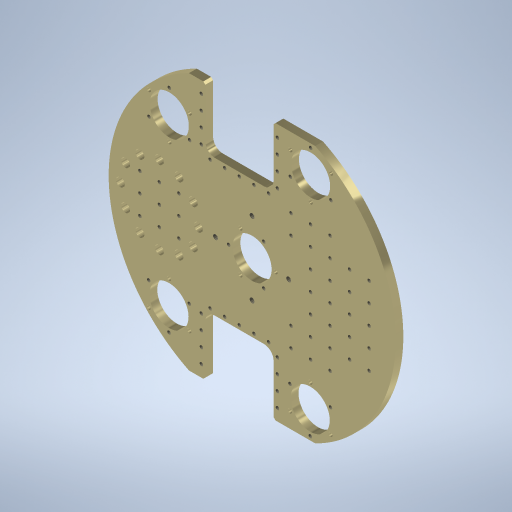
# Autodesk Inventor part: MXC_Plate_drawing
Saved by Autodesk Inventor 2024 (Build 280153000, 153)
## iProperties
Created: 2020-10-08
Part Number: MXC_Plate_drawing
Material: Generic
Document SubType Name: Modeling
Designer: mforsch
Density: 1 g/cm^3
Appearance: Default
Author: mforsch
Autodesk Inventor part; units mm, degrees
ref_plane "YZ Plane" through (0, 0, 0) normal (1, 0, 0) x (0, 1, 0)
ref_plane "XZ Plane" through (0, 0, 0) normal (0, 1, 0) x (-1, 0, 0)
ref_plane "XY Plane" through (0, 0, 0) normal (0, 0, 1) x (1, 0, 0)
sketch "Sketch1" plane through (0, 0, 0) normal (0, 0, 1) x (1, 0, 0)
  circle A0 centre (0, 0) radius 147
  dimension "d0" = 294
  constraints: 1 centre point, 1 coincident
  measures "d0" diameter of A0
extrude "Extrusion1" add sketch "Sketch1" along normal blind 8
sketch "Sketch2" plane through (0, 0, 8) normal (0, 0, 1) x (1, 0, 0)
  line L0 (-102.4138, 132) -> (116.069, 132)
  line L1 (116.069, 132) -> (116.069, 183.5862)
  line L2 (116.069, 183.5862) -> (-102.4138, 183.5862)
  line L3 (-102.4138, 183.5862) -> (-102.4138, 132)
  line L4 (-102.4138, -132) -> (116.069, -132)
  line L5 (116.069, -132) -> (116.069, -180.5517)
  line L6 (116.069, -180.5517) -> (-102.4138, -180.5517)
  line L7 (-102.4138, -180.5517) -> (-102.4138, -132)
  line L8 (-38, -70) -> (12, -70)
  line L9 (22, -80) -> (22, -156.14)
  line L10 (22, -156.14) -> (-48, -156.14)
  line L11 (-48, -156.14) -> (-48, -80)
  line L12 (-38, 70) -> (12, 70)
  line L13 (22, 80) -> (22, 183.7215)
  line L14 (22, 183.7215) -> (-48, 183.7215)
  line L15 (-48, 183.7215) -> (-48, 80)
  arc A0 (-48, 80) -> (-38, 70) centre (-38, 80) ccw
  arc A1 (12, 70) -> (22, 80) centre (12, 80) ccw
  arc A2 (-38, -70) -> (-48, -80) centre (-38, -80) ccw
  arc A3 (22, -80) -> (12, -70) centre (12, -80) ccw
  point P0 (0, 0)
  point P1 (-48, 70)
  dimension "d3" = 264
  dimension "d4" = 132
  dimension "d5" = 70
  dimension "d6" = 70
  dimension "d7" = 22
  dimension "d8" = 48
  dimension "d9" = 10
  dimension "d10" = 10
  dimension "d11" = 10
  constraints: 32 end point, 8 parallel, 8 point on circle, 8 tangent, 6 point on line, 4 centre point, 4 horizontal, 4 perpendicular, 1 equal radius
  measures "d3" distance between parallel lines of L4 L0
  measures "d4" distance from line of point (0, 0) L4
  measures "d5" distance from line of point (0, 0) L12
  measures "d6" distance from line of point (0, 0) L8
  measures "d7" distance from line of point (0, 0) L13
  measures "d8" distance from line of point (0, 0) L15
  measures "d9" radius of A0
  measures "d10" radius of A1
  measures "d11" radius of A2
extrude "Extrusion2" cut sketch "Sketch2" against normal blind 8
chamfer "Chamfer1" distance 2 angle 45 4 edges at (-48, 132, 4) (22, 132, 4) (-48, -132, 4) (22, -132, 4)
sketch "Sketch4" plane through (0, 0, 0) normal (0, 0, -1) x (-1, 0, 0)
  circle A0 centre (0, 0) radius 120
  arc A1 (-64.6916, 132) -> (-64.6916, -132) centre (0, 0) ccw projected
  arc A2 (84.8528, 84.8528) -> (0, 120) centre (0, 0) ccw
  line L0 (0, 0) -> (84.8528, 84.8528) construction
  line L1 (0, 0) -> (0, 120) construction
  arc A3 (0, 120) -> (-60, 103.923) centre (0, 0) ccw
  line L2 (0, 0) -> (-60, 103.923) construction
  line L3 (0, 0) -> (0, 120) construction
  arc A4 (0.4606, -119.9991) -> (85.1779, -84.5265) centre (0, 0) ccw
  line L4 (0, 0) -> (85.1779, -84.5265) construction
  line L5 (0, 0) -> (0.4606, -119.9991) construction
  arc A5 (-59.6006, -104.1526) -> (0.4606, -119.9991) centre (0, 0) ccw
  line L6 (0, 0) -> (-59.6006, -104.1526) construction
  line L7 (0, 0) -> (0.4606, -119.9991) construction
  dimension "d18" = 240
  dimension "d25" = 45
  dimension "d26" = 30
  dimension "d27" = 45
  dimension "d28" = 30
  constraints: 16 end point, 11 point on circle, 10 coincident, 5 centre point
  measures "d18" diameter of A0
  measures "d25" angle of L0 L1
  measures "d26" angle of L3 L2
  measures "d27" angle of L5 L4
  measures "d28" angle of L6 L7
hole "40mm cutouts" at (0, 0, 0) at (60, 103.923, 0) at (-84.8528, 84.8528, 0) at (-85.1779, -84.5265, 0) at (59.6006, -104.1526, 0) direction (0, 0, 1) diameter 40 end through all
sketch "Sketch5" plane through (0, 0, 0) normal (0, 0, -1) x (-1, 0, 0)
  line L0 (0, 0) -> (233.6679, 0)
  line L1 (0, 0) -> (0, 89.9705)
  point P0 (95, 0)
  point P1 (135, 0)
  point P2 (129.641, 20)
  point P3 (115, 34.641)
  point P4 (95, 40)
  point P5 (75, 34.641)
  point P6 (60.359, 20)
  point P7 (55, 0)
  point P8 (60.359, -20)
  point P9 (75, -34.641)
  point P10 (95, -40)
  point P11 (115, -34.641)
  point P12 (129.641, -20)
  dimension "d38" = 360
  dimension "d40" = 40
  constraints: 4 end point, 1 horizontal, 1 vertical, 13 other
  measures "d40" distance of point (135, 0) point (95, 0)
hole "Mixing Chamber Mount" at (-135, 0, 0) at (-129.641, 20, 0) at (-115, 34.641, 0) at (-95, 40, 0) at (-75, 34.641, 0) at (-60.359, 20, 0) at (-55, 0, 0) at (-60.359, -20, 0) at (-75, -34.641, 0) at (-95, -40, 0) at (-115, -34.641, 0) at (-129.641, -20, 0) direction (0, 0, 1) diameter 9 end through all
sketch "Sketch6" plane through (0, 0, 0) normal (0, 0, -1) x (-1, 0, 0)
  line L0 (0, 0) -> (0, 75.3949)
  line L1 (0, 0) -> (40.5445, 0)
  circle A0 centre (-60, 103.923) radius 20 projected
  circle A1 centre (-60, 103.923) radius 24
  circle A2 centre (84.8528, 84.8528) radius 20 projected
  circle A3 centre (84.8528, 84.8528) radius 24
  circle A4 centre (0, 0) radius 24
  circle A5 centre (-59.6006, -104.1526) radius 20 projected
  circle A6 centre (-59.6006, -104.1526) radius 24
  circle A7 centre (85.1779, -84.5265) radius 20 projected
  circle A8 centre (85.1779, -84.5265) radius 24
  point P0 (75, -20)
  point P1 (75, 0)
  point P2 (95, -20)
  point P3 (95, 0)
  point P4 (75, 20)
  point P5 (95, 20)
  point P6 (115, -20)
  point P7 (115, 0)
  point P8 (115, 20)
  point P9 (-60, 40)
  point P10 (-60, 20)
  point P11 (-60, 0)
  point P12 (-60, -20)
  point P13 (-60, -40)
  point P14 (-80, 40)
  point P15 (-80, 20)
  point P16 (-80, 0)
  point P17 (-80, -20)
  point P18 (-80, -40)
  point P19 (-100, 40)
  point P20 (-100, 20)
  point P21 (-100, 0)
  point P22 (-100, -20)
  point P23 (-100, -40)
  point P24 (-120, 40)
  point P25 (-120, 20)
  point P26 (-120, 0)
  point P27 (-120, -20)
  point P28 (-120, -40)
  point P29 (-40, 40)
  point P30 (-40, 60)
  point P31 (-60, 60)
  point P32 (-80, 60)
  point P33 (-40, -40)
  point P34 (-40, -60)
  point P35 (-60, -60)
  point P36 (-80, -60)
  point P37 (-26, -75)
  point P38 (52, -75)
  point P39 (-17, -66)
  point P40 (-2, -66)
  point P41 (13, -66)
  point P42 (28, -66)
  point P43 (43, -66)
  point P44 (-26, -90)
  point P45 (52, -90)
  point P46 (-26, -105)
  point P47 (52, -105)
  point P48 (-26, -120)
  point P49 (52, -120)
  point P50 (-26, 75)
  point P51 (52, 75)
  point P52 (-17, 66)
  point P53 (-2, 66)
  point P54 (13, 66)
  point P55 (28, 66)
  point P56 (43, 66)
  point P57 (-26, 90)
  point P58 (52, 90)
  point P59 (-26, 105)
  point P60 (52, 105)
  point P61 (-26, 120)
  point P62 (52, 120)
  point P63 (-59.6006, -128.1526)
  point P64 (85.1779, -108.5265)
  point P65 (84.8528, 108.8528)
  point P66 (-60, 127.923)
  point P67 (-80.7846, 91.923)
  point P68 (-39.2154, 91.923)
  point P69 (64.0682, 72.8528)
  point P70 (105.6374, 72.8528)
  point P71 (105.9625, -72.5265)
  point P72 (64.3933, -72.5265)
  point P73 (-38.816, -92.1526)
  point P74 (-80.3852, -92.1526)
  point P75 (24, 0)
  point P76 (-12, 20.7846)
  point P77 (-12, -20.7846)
  dimension "d90" = 48
  dimension "d91" = 48
  dimension "d92" = 48
  dimension "d93" = 48
  dimension "d94" = 48
  dimension "d52" = 20
  dimension "d55" = 20
  dimension "d58" = 75
  dimension "d59" = 20
  dimension "d60" = 60
  dimension "d61" = 40
  dimension "d64" = 20
  dimension "d67" = 20
  dimension "d71" = 75
  dimension "d72" = 26
  dimension "d73" = 9
  dimension "d74" = 9
  dimension "d78" = 15
  dimension "d85" = 15
  dimension "d97" = 360
  dimension "d101" = 360
  dimension "d105" = 360
  dimension "d109" = 360
  dimension "d124" = 360
  constraints: 13 symmetric about line, 5 coincident, 4 end point, 4 horizontal, 4 vertical, 4 vertical alignment, 1 horizontal alignment, 1 point on line, 67 other
  measures "d52" distance of point (75, -20) point (75, 0)
  measures "d55" distance of point (75, -20) point (95, -20)
  measures "d58" horizontal distance of point (75, -20) L0.start
  measures "d59" vertical distance of point (75, -20) L0.start
  measures "d60" distance from line of L0 point (-60, 40)
  measures "d61" distance from line of L1 point (-60, 40)
  measures "d64" distance of point (-60, 40) point (-60, 20)
  measures "d67" distance of point (-60, 40) point (-80, 40)
  measures "d71" distance from line of L1 point (-26, -75)
  measures "d72" distance from line of L0 point (-26, -75)
  measures "d73" horizontal distance of point (-17, -66) point (-26, -75)
  measures "d74" horizontal distance of point (-26, -75) point (-17, -66)
  measures "d78" distance of point (-17, -66) point (-2, -66)
  measures "d85" distance of point (-26, -75) point (-26, -90)
hole "M4 mounting holes" at (-75, -20, 0) at (-75, 0, 0) at (-95, -20, 0) at (-95, 0, 0) at (-75, 20, 0) at (-95, 20, 0) at (-115, -20, 0) at (-115, 0, 0) at (-115, 20, 0) at (60, 40, 0) at (60, 20, 0) at (60, 0, 0) at (60, -20, 0) at (60, -40, 0) at (80, 40, 0) at (80, 20, 0) at (80, 0, 0) at (80, -20, 0) at (80, -40, 0) at (100, 40, 0) at (100, 20, 0) at (100, 0, 0) at (100, -20, 0) at (100, -40, 0) at (120, 40, 0) at (120, 20, 0) at (120, 0, 0) at (120, -20, 0) at (120, -40, 0) at (40, 40, 0) at (40, 60, 0) at (60, 60, 0) at (80, 60, 0) at (40, -40, 0) at (40, -60, 0) at (60, -60, 0) at (80, -60, 0) at (26, -75, 0) at (-52, -75, 0) at (17, -66, 0) at (2, -66, 0) at (-13, -66, 0) at (-28, -66, 0) at (-43, -66, 0) at (26, -90, 0) at (-52, -90, 0) at (26, -105, 0) at (-52, -105, 0) at (26, -120, 0) at (-52, -120, 0) direction (0, 0, 1) diameter 3.459 end through all and at (17, 66, 0) (2, 66, 0) (-13, 66, 0) (-28, 66, 0) (-43, 66, 0) (-52, 75, 0) (-52, 90, 0) (26, 75, 0) (26, 90, 0) (26, 105, 0) (26, 120, 0) (-52, 105, 0) (-52, 120, 0) (59.6006, -128.1526, 0) (-85.1779, -108.5265, 0) (-84.8528, 108.8528, 0) (60, 127.923, 0) (80.7846, 91.923, 0) (39.2154, 91.923, 0) (-64.0682, 72.8528, 0) (-105.6374, 72.8528, 0) (-105.9625, -72.5265, 0) (-64.3933, -72.5265, 0) (38.816, -92.1526, 0) (80.3852, -92.1526, 0) (12, 20.7846, 0) (12, -20.7846, 0) (-24, 0, 0) thread size "M4x0.5" class "6H" standard "ANSI Metric M Profile"
sketch "Sketch7" plane through (0, 0, 0) normal (0, 0, -1) x (-1, 0, 0)
  circle A0 centre (0, 0) radius 24
  circle A1 centre (84.8528, 84.8528) radius 20 projected
  circle A2 centre (84.8528, 84.8528) radius 24
  circle A3 centre (-60, 103.923) radius 20 projected
  circle A4 centre (-60, 103.923) radius 24
  circle A5 centre (-59.6006, -104.1526) radius 20 projected
  circle A6 centre (-59.6006, -104.1526) radius 24
  circle A7 centre (85.1779, -84.5265) radius 20 projected
  circle A8 centre (85.1779, -84.5265) radius 24
  point P0 (-24, 0)
  point P1 (84.8528, 60.8528)
  point P2 (-60, 79.923)
  point P3 (-59.6006, -80.1526)
  point P4 (85.1779, -60.5265)
  point P5 (64.3933, -96.5265)
  point P6 (105.9625, -96.5265)
  point P7 (-80.3852, -116.1526)
  point P8 (-38.816, -116.1526)
  point P9 (12, -20.7846)
  point P10 (12, 20.7846)
  point P11 (105.6374, 96.8528)
  point P12 (64.0682, 96.8528)
  point P13 (-39.2154, 115.923)
  point P14 (-80.7846, 115.923)
  dimension "d126" = 48
  dimension "d127" = 48
  dimension "d128" = 48
  dimension "d129" = 48
  dimension "d130" = 48
  dimension "d133" = 360
  dimension "d137" = 360
  dimension "d141" = 360
  dimension "d145" = 360
  dimension "d149" = 360
  constraints: 5 coincident, 4 vertical alignment, 1 horizontal alignment, 30 other
hole "M4 clearance holes" at (24, 0, 0) at (-84.8528, 60.8528, 0) at (60, 79.923, 0) at (59.6006, -80.1526, 0) at (-85.1779, -60.5265, 0) at (-64.3933, -96.5265, 0) at (-105.9625, -96.5265, 0) at (80.3852, -116.1526, 0) at (38.816, -116.1526, 0) at (-12, -20.7846, 0) at (-12, 20.7846, 0) at (-105.6374, 96.8528, 0) at (-64.0682, 96.8528, 0) at (39.2154, 115.923, 0) at (80.7846, 115.923, 0) direction (0, 0, 1) diameter 4.2 end through all
sketch "Sketch8" plane through (0, 0, 0) normal (0, 0, -1) x (-1, 0, 0)
  circle A0 centre (0, 0) radius 37.5
  point P0 (0, 37.5)
  point P1 (-37.5, 0)
  point P2 (0, -37.5)
  point P3 (37.5, 0)
  dimension "d158" = 75
  dimension "d161" = 360
  constraints: 1 coincident, 1 vertical alignment, 7 other
hole "M6 mounting holes" at (0, 37.5, 0) at (37.5, 0, 0) at (0, -37.5, 0) at (-37.5, 0, 0) direction (0, 0, 1) diameter 4.917 end through all thread size "M6x1" class "6H" standard "ANSI Metric M Profile"
body "Solid1"
